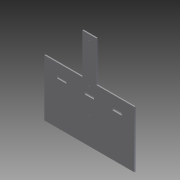
# Autodesk Inventor part: it ftront
Saved by Autodesk Inventor 2011 (Build 150239000, 239)
## iProperties
Created: 2011-08-27
Part Number: it ftront
Document SubType Name: Modeling
Designer: Matthew
Density: 1 g/cm^3
Author: Matthew
Autodesk Inventor part; units mm, degrees
(part 1 of 2)
ref_plane "YZ Plane" through (0, 0, 0) normal (1, 0, 0) x (0, 1, 0)
ref_plane "XZ Plane" through (0, 0, 0) normal (0, 1, 0) x (-1, 0, 0)
ref_plane "XY Plane" through (0, 0, 0) normal (0, 0, 1) x (1, 0, 0)
sketch "Sketch1" plane through (0, 0, 0) normal (0, 0, 1) x (1, 0, 0)
  line L0 (-143.8457, 172.4284) -> (351.4543, 172.4284)
  line L1 (351.4543, 172.4284) -> (351.4543, -716.5716)
  line L2 (351.4543, -716.5716) -> (-143.8457, -716.5716)
  line L3 (-143.8457, -716.5716) -> (-143.8457, 172.4284)
  point P0 (0, 0)
  dimension "d0" = 495.3
  dimension "d1" = 889
  constraints: 8 end point, 2 parallel, 1 horizontal, 1 perpendicular
  measures "d0" distance of L1.end L2.end
  measures "d1" distance of L0.end L1.end
extrude "Extrusion1" add sketch "Sketch1" along normal blind 6.35
sketch "Sketch2" plane through (0, 0, 6.35) normal (0, 0, 1) x (1, 0, 0)
  line L0 (-143.8457, -716.5716) -> (-105.7457, -716.5716)
  line L1 (-105.7457, -716.5716) -> (-105.7457, -640.3716)
  line L2 (-105.7457, -640.3716) -> (-143.8457, -640.3716)
  line L3 (-143.8457, -640.3716) -> (-143.8457, -716.5716)
  line L4 (-105.7457, -640.3716) -> (-124.7957, -640.3716)
  line L5 (-124.7957, -640.3716) -> (-124.7957, -659.4216)
  line L6 (-124.7957, -659.4216) -> (-105.7457, -659.4216)
  line L7 (-105.7457, -659.4216) -> (-105.7457, -640.3716)
  line L8 (351.4543, -716.5716) -> (332.4043, -716.5716)
  line L9 (332.4043, -716.5716) -> (332.4043, -659.4216)
  line L10 (332.4043, -659.4216) -> (351.4543, -659.4216)
  line L11 (351.4543, -659.4216) -> (351.4543, -716.5716)
  circle A0 centre (332.4043, -659.4216) radius 1.9812
  circle A1 centre (-124.7957, -659.4216) radius 1.9812
  point P0 (0, 0)
  dimension "d4" = 38.1
  dimension "d5" = 76.2
  dimension "d6" = 19.05
  dimension "d7" = 19.05
  dimension "d8" = 57.15
  dimension "d9" = 3.9624
  dimension "d10" = 3.9624
  constraints: 24 end point, 6 parallel, 3 horizontal, 3 perpendicular, 2 centre point, 2 coincident
  measures "d4" distance of L2.end L1.end
  measures "d5" distance of L1.end L0.end
  measures "d6" distance of L5.end L4.end
  measures "d7" distance of L9.end L10.end
  measures "d8" distance of L8.end L9.end
  measures "d9" diameter of A0
  measures "d10" diameter of A1
extrude "Extrusion2" cut sketch "Sketch2" against normal blind 6.35 contours A1 L5 L6 | L6 L5 A1 | A0 L10 L9 | L9 L10 A0
sketch "Sketch3" plane through (0, 0, 6.35) normal (0, 0, 1) x (1, 0, 0)
  line L0 (-143.8457, -716.5716) -> (-105.7457, -716.5716)
  line L1 (-105.7457, -716.5716) -> (-105.7457, -640.3716)
  line L2 (-105.7457, -640.3716) -> (-143.8457, -640.3716)
  line L3 (-143.8457, -640.3716) -> (-143.8457, -716.5716)
  line L4 (351.4543, -716.5716) -> (313.3543, -716.5716)
  line L5 (313.3543, -716.5716) -> (313.3543, -640.3716)
  line L6 (313.3543, -640.3716) -> (351.4543, -640.3716)
  line L7 (351.4543, -640.3716) -> (351.4543, -716.5716)
  line L8 (-105.7457, -716.5716) -> (313.3543, -716.5716)
  line L9 (313.3543, -716.5716) -> (313.3543, -691.1716)
  line L10 (313.3543, -691.1716) -> (-105.7457, -691.1716)
  line L11 (-105.7457, -691.1716) -> (-105.7457, -716.5716)
  line L12 (-105.7457, -691.1716) -> (313.3543, -691.1716)
  line L13 (313.3543, -691.1716) -> (313.3543, 127.9784)
  line L14 (313.3543, 127.9784) -> (-105.7457, 127.9784)
  line L15 (-105.7457, 127.9784) -> (-105.7457, -691.1716)
  point P0 (0, 0)
  dimension "d13" = 38.1
  dimension "d14" = 76.2
  dimension "d15" = 38.1
  dimension "d16" = 25.4
  dimension "d17" = 819.15
  constraints: 32 end point, 8 parallel, 4 horizontal, 4 perpendicular, 1 point on line
  measures "d13" distance of L2.end L1.end
  measures "d14" distance of L1.end L0.end
  measures "d15" distance of L5.end L6.end
  measures "d16" distance of L9.end L8.end
  measures "d17" distance of L13.end L12.end
extrude "Extrusion3" cut sketch "Sketch3" against normal blind 6.35 contours L1 L15 L14 L13 L5 L10
sketch "Sketch4" plane through (0, 0, 6.35) normal (0, 0, 1) x (1, 0, 0)
  circle A0 centre (332.4043, -659.4216) radius 1.9812 projected
  circle A1 centre (-124.7957, -659.4216) radius 1.9812 projected
  line L0 (-143.8457, -716.5716) -> (-93.0457, -716.5716)
  line L1 (-93.0457, -716.5716) -> (-93.0457, -627.6716)
  line L2 (-93.0457, -627.6716) -> (-143.8457, -627.6716)
  line L3 (-143.8457, -627.6716) -> (-143.8457, -716.5716)
  line L4 (351.4543, -716.5716) -> (300.6543, -716.5716)
  line L5 (300.6543, -716.5716) -> (300.6543, -627.6716)
  line L6 (300.6543, -627.6716) -> (351.4543, -627.6716)
  line L7 (351.4543, -627.6716) -> (351.4543, -716.5716)
  line L8 (-93.0457, -716.5716) -> (300.6543, -716.5716)
  line L9 (300.6543, -716.5716) -> (300.6543, -678.4716)
  line L10 (300.6543, -678.4716) -> (-93.0457, -678.4716)
  line L11 (-93.0457, -678.4716) -> (-93.0457, -716.5716)
  point P0 (0, 0)
  dimension "d20" = 50.8
  dimension "d21" = 88.9
  dimension "d22" = 50.8
  dimension "d23" = 88.9
  dimension "d24" = 38.1
  constraints: 24 end point, 6 parallel, 3 horizontal, 3 perpendicular, 1 point on line
  measures "d20" distance of L2.end L1.end
  measures "d21" distance of L1.end L0.end
  measures "d22" distance of L5.end L6.end
  measures "d23" distance of L4.end L5.end
  measures "d24" distance of L9.end L8.end
extrude "Extrusion4" add sketch "Sketch4" against normal blind 6.35
fillet "Fillet1" radius 6.35 8 edges at (-93.0457, -678.4716, 3.175) (-93.0457, -627.6716, 3.175) (-105.7457, -627.6716, 3.175) (300.6543, -627.6716, 3.175) (313.3543, -627.6716, 3.175) (300.6543, -678.4716, 3.175) (313.3543, 127.9784, 3.175) (-105.7457, 127.9784, 3.175)
sketch "Sketch5" plane through (0, 0, 6.35) normal (0, 0, 1) x (1, 0, 0)
  line L0 (351.4543, -716.5716) -> (-143.8457, -716.5716) projected
  line L1 (351.4543, -716.5716) -> (345.1043, -716.5716)
  line L2 (345.1043, -716.5716) -> (345.1043, -710.2216)
  line L3 (345.1043, -710.2216) -> (351.4543, -710.2216)
  line L4 (351.4543, -710.2216) -> (351.4543, -716.5716)
  line L5 (345.1043, -710.2216) -> (319.7043, -710.2216)
  line L6 (319.7043, -710.2216) -> (319.7043, -716.5716)
  line L7 (319.7043, -716.5716) -> (345.1043, -716.5716)
  line L8 (345.1043, -716.5716) -> (345.1043, -710.2216)
  line L9 (319.7043, -710.2216) -> (294.3043, -710.2216)
  line L10 (294.3043, -710.2216) -> (294.3043, -716.5716)
  line L11 (294.3043, -716.5716) -> (319.7043, -716.5716)
  line L12 (319.7043, -716.5716) -> (319.7043, -710.2216)
  line L13 (294.3043, -710.2216) -> (268.9043, -710.2216)
  line L14 (268.9043, -710.2216) -> (268.9043, -716.5716)
  line L15 (268.9043, -716.5716) -> (294.3043, -716.5716)
  line L16 (294.3043, -716.5716) -> (294.3043, -710.2216)
  line L17 (268.9043, -710.2216) -> (243.5043, -710.2216)
  line L18 (243.5043, -710.2216) -> (243.5043, -716.5716)
  line L19 (243.5043, -716.5716) -> (268.9043, -716.5716)
  line L20 (268.9043, -716.5716) -> (268.9043, -710.2216)
  line L21 (243.5043, -710.2216) -> (218.1043, -710.2216)
  line L22 (218.1043, -710.2216) -> (218.1043, -716.5716)
  line L23 (218.1043, -716.5716) -> (243.5043, -716.5716)
  line L24 (243.5043, -716.5716) -> (243.5043, -710.2216)
  line L25 (218.1043, -710.2216) -> (192.7043, -710.2216)
  line L26 (192.7043, -710.2216) -> (192.7043, -716.5716)
  line L27 (192.7043, -716.5716) -> (218.1043, -716.5716)
  line L28 (218.1043, -716.5716) -> (218.1043, -710.2216)
  line L29 (192.7043, -710.2216) -> (167.3043, -710.2216)
  line L30 (167.3043, -710.2216) -> (167.3043, -716.5716)
  line L31 (167.3043, -716.5716) -> (192.7043, -716.5716)
  line L32 (192.7043, -716.5716) -> (192.7043, -710.2216)
  line L33 (167.3043, -710.2216) -> (141.9043, -710.2216)
  line L34 (141.9043, -710.2216) -> (141.9043, -716.5716)
  line L35 (141.9043, -716.5716) -> (167.3043, -716.5716)
  line L36 (167.3043, -716.5716) -> (167.3043, -710.2216)
  line L37 (141.9043, -710.2216) -> (116.5043, -710.2216)
  line L38 (116.5043, -710.2216) -> (116.5043, -716.5716)
  line L39 (116.5043, -716.5716) -> (141.9043, -716.5716)
  line L40 (141.9043, -716.5716) -> (141.9043, -710.2216)
  line L41 (116.5043, -710.2216) -> (91.1043, -710.2216)
  line L42 (91.1043, -710.2216) -> (91.1043, -716.5716)
  line L43 (91.1043, -716.5716) -> (116.5043, -716.5716)
  line L44 (116.5043, -716.5716) -> (116.5043, -710.2216)
  line L45 (91.1043, -710.2216) -> (65.7043, -710.2216)
  line L46 (65.7043, -710.2216) -> (65.7043, -716.5716)
  line L47 (65.7043, -716.5716) -> (91.1043, -716.5716)
  line L48 (91.1043, -716.5716) -> (91.1043, -710.2216)
  line L49 (65.7043, -710.2216) -> (40.3043, -710.2216)
  line L50 (40.3043, -710.2216) -> (40.3043, -716.5716)
  line L51 (40.3043, -716.5716) -> (65.7043, -716.5716)
  line L52 (65.7043, -716.5716) -> (65.7043, -710.2216)
  line L53 (40.3043, -710.2216) -> (14.9043, -710.2216)
  line L54 (14.9043, -710.2216) -> (14.9043, -716.5716)
  line L55 (14.9043, -716.5716) -> (40.3043, -716.5716)
  line L56 (40.3043, -716.5716) -> (40.3043, -710.2216)
  line L57 (14.9043, -710.2216) -> (-10.4957, -710.2216)
  line L58 (-10.4957, -710.2216) -> (-10.4957, -716.5716)
  line L59 (-10.4957, -716.5716) -> (14.9043, -716.5716)
  line L60 (14.9043, -716.5716) -> (14.9043, -710.2216)
  line L61 (-10.4957, -710.2216) -> (-35.8957, -710.2216)
  line L62 (-35.8957, -710.2216) -> (-35.8957, -716.5716)
  line L63 (-35.8957, -716.5716) -> (-10.4957, -716.5716)
  line L64 (-10.4957, -716.5716) -> (-10.4957, -710.2216)
  line L65 (-35.8957, -710.2216) -> (-61.2957, -710.2216)
  line L66 (-61.2957, -710.2216) -> (-61.2957, -716.5716)
  line L67 (-61.2957, -716.5716) -> (-35.8957, -716.5716)
  line L68 (-35.8957, -716.5716) -> (-35.8957, -710.2216)
  line L69 (-61.2957, -710.2216) -> (-86.6957, -710.2216)
  line L70 (-86.6957, -710.2216) -> (-86.6957, -716.5716)
  line L71 (-86.6957, -716.5716) -> (-61.2957, -716.5716)
  line L72 (-61.2957, -716.5716) -> (-61.2957, -710.2216)
  line L73 (-86.6957, -710.2216) -> (-112.0957, -710.2216)
  line L74 (-112.0957, -710.2216) -> (-112.0957, -716.5716)
  line L75 (-112.0957, -716.5716) -> (-86.6957, -716.5716)
  line L76 (-86.6957, -716.5716) -> (-86.6957, -710.2216)
  line L77 (-112.0957, -710.2216) -> (-137.4957, -710.2216)
  line L78 (-137.4957, -710.2216) -> (-137.4957, -716.5716)
  line L79 (-137.4957, -716.5716) -> (-112.0957, -716.5716)
  line L80 (-112.0957, -716.5716) -> (-112.0957, -710.2216)
  point P0 (0, 0)
  dimension "d28" = 6.35
  dimension "d29" = 6.35
  dimension "d30" = 25.4
  dimension "d31" = 25.4
  dimension "d32" = 25.4
  dimension "d33" = 25.4
  dimension "d34" = 25.4
  dimension "d35" = 25.4
  dimension "d36" = 25.4
  dimension "d37" = 25.4
  dimension "d38" = 25.4
  dimension "d39" = 25.4
  dimension "d40" = 25.4
  dimension "d41" = 25.4
  dimension "d42" = 25.4
  dimension "d43" = 25.4
  dimension "d44" = 25.4
  dimension "d45" = 25.4
  dimension "d46" = 25.4
  dimension "d47" = 25.4
  dimension "d48" = 25.4
  constraints: 160 end point, 40 parallel, 20 horizontal, 20 perpendicular, 20 other
  measures "d28" distance of L2.end L3.end
  measures "d29" distance of L1.end L2.end
  measures "d30" distance of L7.end L6.end
  measures "d31" distance of L11.end L10.end
  measures "d32" distance of L15.end L14.end
  measures "d33" distance of L19.end L18.end
  measures "d34" distance of L23.end L22.end
  measures "d35" distance of L27.end L26.end
  measures "d36" distance of L31.end L30.end
  measures "d37" distance of L35.end L34.end
  measures "d38" distance of L39.end L38.end
  measures "d39" distance of L43.end L42.end
  measures "d40" distance of L47.end L46.end
  measures "d41" distance of L51.end L50.end
  measures "d42" distance of L55.end L54.end
  measures "d43" distance of L59.end L58.end
  measures "d44" distance of L63.end L62.end
  measures "d45" distance of L67.end L66.end
  measures "d46" distance of L71.end L70.end
  measures "d47" distance of L75.end L74.end
  measures "d48" distance of L79.end L78.end
extrude "Extrusion5" cut sketch "Sketch5" against normal blind 6.35 contours L0 L6 L5 L2 | L0 L14 L13 L10 | L0 L22 L21 L18 | L0 L30 L29 L26 | L0 L38 L37 L34 | L0 L46 L45 L42 | L0 L54 L53 L50 | L0 L62 L61 L58 | L0 L70 L69 L66 | L0 L78 L77 L74
sketch "Sketch6" plane through (0, 0, 6.35) normal (0, 0, 1) x (1, 0, 0)
  line L0 (-143.8457, -716.5716) -> (-143.8457, 172.4284) projected
  line L1 (-143.8457, 172.4284) -> (-137.4957, 172.4284)
  line L2 (-137.4957, 172.4284) -> (-137.4957, 121.6284)
  line L3 (-137.4957, 121.6284) -> (-143.8457, 121.6284)
  line L4 (-143.8457, 121.6284) -> (-143.8457, 172.4284)
  line L5 (-137.4957, 121.6284) -> (-143.8457, 121.6284)
  line L6 (-143.8457, 121.6284) -> (-143.8457, 70.8284)
  line L7 (-143.8457, 70.8284) -> (-137.4957, 70.8284)
  line L8 (-137.4957, 70.8284) -> (-137.4957, 121.6284)
  line L9 (-137.4957, 70.8284) -> (-143.8457, 70.8284)
  line L10 (-143.8457, 70.8284) -> (-143.8457, 20.0284)
  line L11 (-143.8457, 20.0284) -> (-137.4957, 20.0284)
  line L12 (-137.4957, 20.0284) -> (-137.4957, 70.8284)
  line L13 (-137.4957, 20.0284) -> (-143.8457, 20.0284)
  line L14 (-143.8457, 20.0284) -> (-143.8457, -30.7716)
  line L15 (-143.8457, -30.7716) -> (-137.4957, -30.7716)
  line L16 (-137.4957, -30.7716) -> (-137.4957, 20.0284)
  line L17 (-137.4957, -30.7716) -> (-143.8457, -30.7716)
  line L18 (-143.8457, -30.7716) -> (-143.8457, -81.5716)
  line L19 (-143.8457, -81.5716) -> (-137.4957, -81.5716)
  line L20 (-137.4957, -81.5716) -> (-137.4957, -30.7716)
  line L21 (-137.4957, -81.5716) -> (-143.8457, -81.5716)
  line L22 (-143.8457, -81.5716) -> (-143.8457, -132.3716)
  line L23 (-143.8457, -132.3716) -> (-137.4957, -132.3716)
  line L24 (-137.4957, -132.3716) -> (-137.4957, -81.5716)
  line L25 (-137.4957, -132.3716) -> (-143.8457, -132.3716)
  line L26 (-143.8457, -132.3716) -> (-143.8457, -183.1716)
  line L27 (-143.8457, -183.1716) -> (-137.4957, -183.1716)
  line L28 (-137.4957, -183.1716) -> (-137.4957, -132.3716)
  line L29 (-137.4957, -183.1716) -> (-143.8457, -183.1716)
  line L30 (-143.8457, -183.1716) -> (-143.8457, -233.9716)
  line L31 (-143.8457, -233.9716) -> (-137.4957, -233.9716)
  line L32 (-137.4957, -233.9716) -> (-137.4957, -183.1716)
  line L33 (-137.4957, -233.9716) -> (-143.8457, -233.9716)
  line L34 (-143.8457, -233.9716) -> (-143.8457, -284.7716)
  line L35 (-143.8457, -284.7716) -> (-137.4957, -284.7716)
  line L36 (-137.4957, -284.7716) -> (-137.4957, -233.9716)
  line L37 (-137.4957, -284.7716) -> (-143.8457, -284.7716)
  line L38 (-143.8457, -284.7716) -> (-143.8457, -335.5716)
  line L39 (-143.8457, -335.5716) -> (-137.4957, -335.5716)
  line L40 (-137.4957, -335.5716) -> (-137.4957, -284.7716)
  line L41 (-137.4957, -335.5716) -> (-143.8457, -335.5716)
  line L42 (-143.8457, -335.5716) -> (-143.8457, -386.3716)
  line L43 (-143.8457, -386.3716) -> (-137.4957, -386.3716)
  line L44 (-137.4957, -386.3716) -> (-137.4957, -335.5716)
  line L45 (-137.4957, -386.3716) -> (-143.8457, -386.3716)
  line L46 (-143.8457, -386.3716) -> (-143.8457, -437.1716)
  line L47 (-143.8457, -437.1716) -> (-137.4957, -437.1716)
  line L48 (-137.4957, -437.1716) -> (-137.4957, -386.3716)
  line L49 (-137.4957, -437.1716) -> (-143.8457, -437.1716)
  line L50 (-143.8457, -437.1716) -> (-143.8457, -487.9716)
  line L51 (-143.8457, -487.9716) -> (-137.4957, -487.9716)
  line L52 (-137.4957, -487.9716) -> (-137.4957, -437.1716)
  line L53 (-137.4957, -487.9716) -> (-143.8457, -487.9716)
  line L54 (-143.8457, -487.9716) -> (-143.8457, -538.7716)
  line L55 (-143.8457, -538.7716) -> (-137.4957, -538.7716)
  line L56 (-137.4957, -538.7716) -> (-137.4957, -487.9716)
  line L57 (-137.4957, -538.7716) -> (-143.8457, -538.7716)
  line L58 (-143.8457, -538.7716) -> (-143.8457, -589.5716)
  line L59 (-143.8457, -589.5716) -> (-137.4957, -589.5716)
  line L60 (-137.4957, -589.5716) -> (-137.4957, -538.7716)
  line L61 (-137.4957, -589.5716) -> (-143.8457, -589.5716)
  line L62 (-143.8457, -589.5716) -> (-143.8457, -640.3716)
  line L63 (-143.8457, -640.3716) -> (-137.4957, -640.3716)
  line L64 (-137.4957, -640.3716) -> (-137.4957, -589.5716)
  line L65 (-137.4957, -640.3716) -> (-143.8457, -640.3716)
  line L66 (-143.8457, -640.3716) -> (-143.8457, -691.1716)
  line L67 (-143.8457, -691.1716) -> (-137.4957, -691.1716)
  line L68 (-137.4957, -691.1716) -> (-137.4957, -640.3716)
  point P0 (0, 0)
  dimension "d51" = 50.8
  dimension "d52" = 50.8
  dimension "d53" = 50.8
  dimension "d54" = 50.8
  dimension "d55" = 50.8
  dimension "d56" = 50.8
  dimension "d57" = 50.8
  dimension "d58" = 50.8
  dimension "d59" = 50.8
  dimension "d60" = 50.8
  dimension "d61" = 50.8
  dimension "d62" = 50.8
  dimension "d63" = 50.8
  dimension "d64" = 50.8
  dimension "d65" = 50.8
  dimension "d66" = 50.8
  dimension "d67" = 50.8
  constraints: 136 end point, 34 parallel, 17 horizontal, 17 perpendicular, 17 other
  measures "d51" distance of L1.end L2.end
  measures "d52" distance of L6.end L5.end
  measures "d53" distance of L10.end L9.end
  measures "d54" distance of L14.end L13.end
  measures "d55" distance of L18.end L17.end
  measures "d56" distance of L22.end L21.end
  measures "d57" distance of L26.end L25.end
  measures "d58" distance of L30.end L29.end
  measures "d59" distance of L34.end L33.end
  measures "d60" distance of L38.end L37.end
  measures "d61" distance of L42.end L41.end
  measures "d62" distance of L46.end L45.end
  measures "d63" distance of L50.end L49.end
  measures "d64" distance of L54.end L53.end
  measures "d65" distance of L58.end L57.end
  measures "d66" distance of L62.end L61.end
  measures "d67" distance of L66.end L65.end
extrude "Extrusion6" cut sketch "Sketch6" against normal blind 6.35 contours L0 L59 L64 L63 | L0 L51 L56 L55 | L0 L43 L48 L47 | L0 L35 L40 L39 | L0 L27 L32 L31 | L0 L19 L24 L23 | L0 L11 L16 L15 | L0 L3 L8 L7
sketch "Sketch7" plane through (0, 0, 6.35) normal (0, 0, 1) x (1, 0, 0)
  line L0 (351.4543, 172.4284) -> (351.4543, -716.5716) projected
  line L1 (-137.4957, 121.6284) -> (351.4543, 121.6284)
  line L2 (-143.8457, 70.8284) -> (351.4543, 70.8284)
  line L3 (351.4543, 121.6284) -> (345.1043, 121.6284)
  line L4 (345.1043, 121.6284) -> (345.1043, 70.8284)
  line L5 (345.1043, 70.8284) -> (351.4543, 70.8284)
  line L6 (351.4543, 70.8284) -> (351.4543, 121.6284)
  line L7 (351.4543, 20.0284) -> (345.1043, 20.0284)
  line L8 (345.1043, 20.0284) -> (345.1043, -30.7716)
  line L9 (345.1043, -30.7716) -> (351.4543, -30.7716)
  line L10 (351.4543, -30.7716) -> (351.4543, 20.0284)
  line L11 (351.4543, -81.5716) -> (345.1043, -81.5716)
  line L12 (345.1043, -81.5716) -> (345.1043, -132.3716)
  line L13 (345.1043, -132.3716) -> (351.4543, -132.3716)
  line L14 (351.4543, -132.3716) -> (351.4543, -81.5716)
  line L15 (351.4543, -183.1716) -> (345.1043, -183.1716)
  line L16 (345.1043, -183.1716) -> (345.1043, -233.9716)
  line L17 (345.1043, -233.9716) -> (351.4543, -233.9716)
  line L18 (351.4543, -233.9716) -> (351.4543, -183.1716)
  line L19 (351.4543, -284.7716) -> (345.1043, -284.7716)
  line L20 (345.1043, -284.7716) -> (345.1043, -335.5716)
  line L21 (345.1043, -335.5716) -> (351.4543, -335.5716)
  line L22 (351.4543, -335.5716) -> (351.4543, -284.7716)
  line L23 (351.4543, -386.3716) -> (345.1043, -386.3716)
  line L24 (345.1043, -386.3716) -> (345.1043, -437.1716)
  line L25 (345.1043, -437.1716) -> (351.4543, -437.1716)
  line L26 (351.4543, -437.1716) -> (351.4543, -386.3716)
  line L27 (351.4543, -487.9716) -> (345.1043, -487.9716)
  line L28 (345.1043, -487.9716) -> (345.1043, -538.7716)
  line L29 (345.1043, -538.7716) -> (351.4543, -538.7716)
  line L30 (351.4543, -538.7716) -> (351.4543, -487.9716)
  line L31 (351.4543, -589.5716) -> (345.1043, -589.5716)
  line L32 (345.1043, -589.5716) -> (345.1043, -640.3716)
  line L33 (345.1043, -640.3716) -> (351.4543, -640.3716)
  line L34 (351.4543, -640.3716) -> (351.4543, -589.5716)
  point P0 (0, 0)
  constraints: 68 end point, 16 parallel, 10 horizontal, 8 perpendicular, 1 point on line, 10 other
extrude "Extrusion7" cut sketch "Sketch7" against normal blind 6.35
sketch "Sketch8" plane through (0, 0, 6.35) normal (0, 0, 1) x (1, 0, 0)
  line L0 (345.1043, -81.5716) -> (351.4543, -81.5716) projected
  line L1 (351.4543, -30.7716) -> (351.4543, -81.5716) projected
  line L2 (351.4543, -30.7716) -> (345.1043, -30.7716) projected
  line L3 (345.1043, -30.7716) -> (345.1043, 20.0284) projected
  line L4 (345.1043, 20.0284) -> (351.4543, 20.0284) projected
  line L5 (351.4543, 70.8284) -> (351.4543, 20.0284) projected
  line L6 (351.4543, 70.8284) -> (345.1043, 70.8284) projected
  line L7 (345.1043, 70.8284) -> (345.1043, 121.6284) projected
  line L8 (345.1043, 121.6284) -> (351.4543, 121.6284) projected
  line L9 (351.4543, 172.4284) -> (351.4543, 121.6284) projected
  line L10 (-143.8457, 172.4284) -> (351.4543, 172.4284) projected
  line L11 (-143.8457, 121.6284) -> (-143.8457, 172.4284) projected
  line L12 (-143.8457, 121.6284) -> (-137.4957, 121.6284) projected
  line L13 (-137.4957, 121.6284) -> (-137.4957, 70.8284) projected
  line L14 (-137.4957, 70.8284) -> (-143.8457, 70.8284) projected
  line L15 (-143.8457, 20.0284) -> (-143.8457, 70.8284) projected
  line L16 (-143.8457, 20.0284) -> (-137.4957, 20.0284) projected
  line L17 (-137.4957, 20.0284) -> (-137.4957, -30.7716) projected
  line L18 (-137.4957, -30.7716) -> (-143.8457, -30.7716) projected
  line L19 (-143.8457, -81.5716) -> (-143.8457, -30.7716) projected
  line L20 (-143.8457, -81.5716) -> (-137.4957, -81.5716) projected
  line L21 (-137.4957, -81.5716) -> (-137.4957, -132.3716) projected
  line L22 (-137.4957, -132.3716) -> (-143.8457, -132.3716) projected
  line L23 (-143.8457, -183.1716) -> (-143.8457, -132.3716) projected
  line L24 (-143.8457, -183.1716) -> (-137.4957, -183.1716) projected
  line L25 (-137.4957, -183.1716) -> (-137.4957, -233.9716) projected
  line L26 (-137.4957, -233.9716) -> (-143.8457, -233.9716) projected
  line L27 (-143.8457, -284.7716) -> (-143.8457, -233.9716) projected
  line L28 (-143.8457, -284.7716) -> (-137.4957, -284.7716) projected
  line L29 (-137.4957, -284.7716) -> (-137.4957, -335.5716) projected
  line L30 (-137.4957, -335.5716) -> (-143.8457, -335.5716) projected
  line L31 (-143.8457, -386.3716) -> (-143.8457, -335.5716) projected
  line L32 (-143.8457, -386.3716) -> (-137.4957, -386.3716) projected
  line L33 (-137.4957, -386.3716) -> (-137.4957, -437.1716) projected
  line L34 (-137.4957, -437.1716) -> (-143.8457, -437.1716) projected
  line L35 (-143.8457, -487.9716) -> (-143.8457, -437.1716) projected
  line L36 (-143.8457, -487.9716) -> (-137.4957, -487.9716) projected
  line L37 (-137.4957, -487.9716) -> (-137.4957, -538.7716) projected
  line L38 (-137.4957, -538.7716) -> (-143.8457, -538.7716) projected
  line L39 (-143.8457, -589.5716) -> (-143.8457, -538.7716) projected
  line L40 (-143.8457, -589.5716) -> (-137.4957, -589.5716) projected
  line L41 (-137.4957, -589.5716) -> (-137.4957, -640.3716) projected
  line L42 (-137.4957, -640.3716) -> (-143.8457, -640.3716) projected
  line L43 (-143.8457, -716.5716) -> (-143.8457, -640.3716) projected
  line L44 (-137.4957, -716.5716) -> (-143.8457, -716.5716) projected
  line L45 (-137.4957, -716.5716) -> (-137.4957, -710.2216) projected
  line L46 (-137.4957, -710.2216) -> (-112.0957, -710.2216) projected
  line L47 (-112.0957, -710.2216) -> (-112.0957, -716.5716) projected
  line L48 (-86.6957, -716.5716) -> (-112.0957, -716.5716) projected
  line L49 (-86.6957, -716.5716) -> (-86.6957, -710.2216) projected
  line L50 (-86.6957, -710.2216) -> (-61.2957, -710.2216) projected
  line L51 (-61.2957, -710.2216) -> (-61.2957, -716.5716) projected
  line L52 (-35.8957, -716.5716) -> (-61.2957, -716.5716) projected
  line L53 (-35.8957, -716.5716) -> (-35.8957, -710.2216) projected
  line L54 (-35.8957, -710.2216) -> (-10.4957, -710.2216) projected
  line L55 (-10.4957, -710.2216) -> (-10.4957, -716.5716) projected
  line L56 (14.9043, -716.5716) -> (-10.4957, -716.5716) projected
  line L57 (14.9043, -716.5716) -> (14.9043, -710.2216) projected
  line L58 (14.9043, -710.2216) -> (40.3043, -710.2216) projected
  line L59 (40.3043, -710.2216) -> (40.3043, -716.5716) projected
  line L60 (65.7043, -716.5716) -> (40.3043, -716.5716) projected
  line L61 (65.7043, -716.5716) -> (65.7043, -710.2216) projected
  line L62 (65.7043, -710.2216) -> (91.1043, -710.2216) projected
  line L63 (91.1043, -710.2216) -> (91.1043, -716.5716) projected
  line L64 (116.5043, -716.5716) -> (91.1043, -716.5716) projected
  line L65 (116.5043, -716.5716) -> (116.5043, -710.2216) projected
  line L66 (116.5043, -710.2216) -> (141.9043, -710.2216) projected
  line L67 (141.9043, -710.2216) -> (141.9043, -716.5716) projected
  line L68 (167.3043, -716.5716) -> (141.9043, -716.5716) projected
  line L69 (167.3043, -716.5716) -> (167.3043, -710.2216) projected
  line L70 (167.3043, -710.2216) -> (192.7043, -710.2216) projected
  line L71 (192.7043, -710.2216) -> (192.7043, -716.5716) projected
  line L72 (218.1043, -716.5716) -> (192.7043, -716.5716) projected
  line L73 (218.1043, -716.5716) -> (218.1043, -710.2216) projected
  line L74 (218.1043, -710.2216) -> (243.5043, -710.2216) projected
  line L75 (243.5043, -710.2216) -> (243.5043, -716.5716) projected
  line L76 (268.9043, -716.5716) -> (243.5043, -716.5716) projected
  line L77 (268.9043, -716.5716) -> (268.9043, -710.2216) projected
  line L78 (268.9043, -710.2216) -> (294.3043, -710.2216) projected
  line L79 (294.3043, -710.2216) -> (294.3043, -716.5716) projected
  line L80 (319.7043, -716.5716) -> (294.3043, -716.5716) projected
  line L81 (319.7043, -716.5716) -> (319.7043, -710.2216) projected
  line L82 (319.7043, -710.2216) -> (345.1043, -710.2216) projected
  line L83 (345.1043, -710.2216) -> (345.1043, -716.5716) projected
  line L84 (351.4543, -716.5716) -> (345.1043, -716.5716) projected
  line L85 (351.4543, -640.3716) -> (351.4543, -716.5716) projected
  line L86 (351.4543, -640.3716) -> (345.1043, -640.3716) projected
  line L87 (345.1043, -640.3716) -> (345.1043, -589.5716) projected
  line L88 (345.1043, -589.5716) -> (351.4543, -589.5716) projected
  line L89 (351.4543, -538.7716) -> (351.4543, -589.5716) projected
  line L90 (351.4543, -538.7716) -> (345.1043, -538.7716) projected
  line L91 (345.1043, -538.7716) -> (345.1043, -487.9716) projected
  line L92 (345.1043, -487.9716) -> (351.4543, -487.9716) projected
  line L93 (351.4543, -437.1716) -> (351.4543, -487.9716) projected
  line L94 (351.4543, -437.1716) -> (345.1043, -437.1716) projected
  line L95 (345.1043, -437.1716) -> (345.1043, -386.3716) projected
  line L96 (345.1043, -386.3716) -> (351.4543, -386.3716) projected
  line L97 (351.4543, -335.5716) -> (351.4543, -386.3716) projected
  line L98 (351.4543, -335.5716) -> (345.1043, -335.5716) projected
  line L99 (345.1043, -335.5716) -> (345.1043, -284.7716) projected
  line L100 (345.1043, -284.7716) -> (351.4543, -284.7716) projected
  line L101 (351.4543, -233.9716) -> (351.4543, -284.7716) projected
  line L102 (351.4543, -233.9716) -> (345.1043, -233.9716) projected
  line L103 (345.1043, -233.9716) -> (345.1043, -183.1716) projected
  line L104 (345.1043, -183.1716) -> (351.4543, -183.1716) projected
  line L105 (351.4543, -132.3716) -> (351.4543, -183.1716) projected
  line L106 (351.4543, -132.3716) -> (345.1043, -132.3716) projected
  line L107 (345.1043, -132.3716) -> (345.1043, -81.5716) projected
  line L108 (313.3543, 121.6284) -> (313.3543, -621.3216) projected
  line L109 (-137.4957, -716.5716) -> (345.1043, -716.5716)
  point P0 (0, 0)
  constraints: 2 end point, 1 perpendicular
extrude "Extrusion8" add sketch "Sketch8" against normal blind 6.35 contours L109 L81 L82 L83 | L109 L77 L78 L79 | L109 L73 L74 L75 | L109 L69 L70 L71 | L109 L65 L66 L67 | L109 L61 L62 L63 | L109 L57 L58 L59 | L109 L53 L54 L55 | L109 L49 L50 L51 | L109 L45 L46 L47
sketch "Sketch9" plane through (0, 0, 6.35) normal (0, 0, 1) x (1, 0, 0)
  line L0 (351.4543, -716.5716) -> (-143.8457, -716.5716) projected
  line L1 (-143.8457, -716.5716) -> (-124.7957, -716.5716)
  line L2 (-124.7957, -716.5716) -> (-124.7957, -710.2216)
  line L3 (-124.7957, -710.2216) -> (-143.8457, -710.2216)
  line L4 (-143.8457, -710.2216) -> (-143.8457, -716.5716)
  line L5 (351.4543, -716.5716) -> (332.4043, -716.5716)
  line L6 (332.4043, -716.5716) -> (332.4043, -710.2216)
  line L7 (332.4043, -710.2216) -> (351.4543, -710.2216)
  line L8 (351.4543, -710.2216) -> (351.4543, -716.5716)
  line L9 (-124.7957, -710.2216) -> (-73.9957, -710.2216)
  line L10 (-73.9957, -710.2216) -> (-73.9957, -716.5716)
  line L11 (-73.9957, -716.5716) -> (-124.7957, -716.5716)
  line L12 (-124.7957, -716.5716) -> (-124.7957, -710.2216)
  line L13 (-73.9957, -710.2216) -> (-23.1957, -710.2216)
  line L14 (-23.1957, -710.2216) -> (-23.1957, -716.5716)
  line L15 (-23.1957, -716.5716) -> (-73.9957, -716.5716)
  line L16 (-73.9957, -716.5716) -> (-73.9957, -710.2216)
  line L17 (-23.1957, -710.2216) -> (27.6043, -710.2216)
  line L18 (27.6043, -710.2216) -> (27.6043, -716.5716)
  line L19 (27.6043, -716.5716) -> (-23.1957, -716.5716)
  line L20 (-23.1957, -716.5716) -> (-23.1957, -710.2216)
  line L21 (27.6043, -710.2216) -> (78.4043, -710.2216)
  line L22 (78.4043, -710.2216) -> (78.4043, -716.5716)
  line L23 (78.4043, -716.5716) -> (27.6043, -716.5716)
  line L24 (27.6043, -716.5716) -> (27.6043, -710.2216)
  line L25 (78.4043, -716.5716) -> (129.2043, -716.5716)
  line L26 (129.2043, -716.5716) -> (129.2043, -710.2216)
  line L27 (129.2043, -710.2216) -> (78.4043, -710.2216)
  line L28 (78.4043, -710.2216) -> (78.4043, -716.5716)
  line L29 (129.2043, -710.2216) -> (180.0043, -710.2216)
  line L30 (180.0043, -710.2216) -> (180.0043, -716.5716)
  line L31 (180.0043, -716.5716) -> (129.2043, -716.5716)
  line L32 (129.2043, -716.5716) -> (129.2043, -710.2216)
  line L33 (180.0043, -716.5716) -> (230.8043, -716.5716)
  line L34 (230.8043, -716.5716) -> (230.8043, -710.2216)
  line L35 (230.8043, -710.2216) -> (180.0043, -710.2216)
  line L36 (180.0043, -710.2216) -> (180.0043, -716.5716)
  line L37 (230.8043, -710.2216) -> (281.6043, -710.2216)
  line L38 (281.6043, -710.2216) -> (281.6043, -716.5716)
  line L39 (281.6043, -716.5716) -> (230.8043, -716.5716)
  line L40 (230.8043, -716.5716) -> (230.8043, -710.2216)
  line L41 (281.6043, -710.2216) -> (332.4043, -710.2216)
  line L42 (332.4043, -710.2216) -> (332.4043, -716.5716)
  line L43 (332.4043, -716.5716) -> (281.6043, -716.5716)
  line L44 (281.6043, -716.5716) -> (281.6043, -710.2216)
  point P0 (0, 0)
  dimension "d74" = 19.05
  dimension "d75" = 6.35
  dimension "d76" = 19.05
  dimension "d77" = 6.35
  dimension "d78" = 50.8
  dimension "d79" = 50.8
  dimension "d80" = 50.8
  dimension "d81" = 50.8
  dimension "d82" = 50.8
  dimension "d83" = 50.8
  dimension "d84" = 50.8
  dimension "d85" = 50.8
  constraints: 88 end point, 22 parallel, 11 horizontal, 11 perpendicular, 6 point on line
  measures "d74" distance of L3.end L2.end
  measures "d75" distance of L2.end L1.end
  measures "d76" distance of L6.end L7.end
  measures "d77" distance of L5.end L6.end
  measures "d78" distance of L10.end L11.end
  measures "d79" distance of L14.end L15.end
  measures "d80" distance of L18.end L19.end
  measures "d81" distance of L22.end L23.end
  measures "d82" distance of L27.end L26.end
  measures "d83" distance of L30.end L31.end
  measures "d84" distance of L35.end L34.end
  measures "d85" distance of L38.end L39.end
extrude "Extrusion9" cut sketch "Sketch9" against normal blind 6.35 contours L0 L38 L41 L6 | L0 L14 L17 L18
sketch "Sketch10" plane through (0, 0, 6.35) normal (0, 0, 1) x (1, 0, 0)
  line L0 (281.6043, -716.5716) -> (27.6043, -716.5716) projected
  line L1 (-23.1957, -716.5716) -> (-143.8457, -716.5716) projected
  line L2 (-23.1957, -716.5716) -> (-73.9957, -716.5716)
  line L3 (-73.9957, -716.5716) -> (-73.9957, -710.2216)
  line L4 (-73.9957, -710.2216) -> (-23.1957, -710.2216)
  line L5 (-23.1957, -710.2216) -> (-23.1957, -716.5716)
  line L6 (-73.9957, -710.2216) -> (-124.7957, -710.2216)
  line L7 (-124.7957, -710.2216) -> (-124.7957, -716.5716)
  line L8 (-124.7957, -716.5716) -> (-73.9957, -716.5716)
  line L9 (-73.9957, -716.5716) -> (-73.9957, -710.2216)
  line L10 (27.6043, -710.2216) -> (78.4043, -710.2216)
  line L11 (78.4043, -710.2216) -> (78.4043, -716.5716)
  line L12 (78.4043, -716.5716) -> (27.6043, -716.5716)
  line L13 (27.6043, -716.5716) -> (27.6043, -710.2216)
  line L14 (78.4043, -710.2216) -> (129.2043, -710.2216)
  line L15 (129.2043, -710.2216) -> (129.2043, -716.5716)
  line L16 (129.2043, -716.5716) -> (78.4043, -716.5716)
  line L17 (78.4043, -716.5716) -> (78.4043, -710.2216)
  point P0 (0, 0)
  dimension "d88" = 50.8
  dimension "d89" = 50.8
  dimension "d90" = 50.8
  dimension "d91" = 50.8
  constraints: 32 end point, 8 parallel, 4 horizontal, 4 perpendicular, 3 point on line
  measures "d88" distance of L3.end L4.end
  measures "d89" distance of L8.end L7.end
  measures "d90" distance of L11.end L12.end
  measures "d91" distance of L15.end L16.end
extrude "Extrusion10" cut sketch "Sketch10" against normal blind 6.35 contours L0 L11 L14 L15 | L1 L7 L6 L3
sketch "Sketch11" plane through (0, 0, 6.35) normal (0, 0, 1) x (1, 0, 0)
  line L0 (281.6043, -716.5716) -> (129.2043, -716.5716) projected
  line L1 (129.2043, -710.2216) -> (180.0043, -710.2216)
  line L2 (180.0043, -710.2216) -> (180.0043, -716.5716)
  line L3 (180.0043, -716.5716) -> (129.2043, -716.5716)
  line L4 (129.2043, -716.5716) -> (129.2043, -710.2216)
  line L5 (180.0043, -710.2216) -> (230.8043, -710.2216)
  line L6 (230.8043, -710.2216) -> (230.8043, -716.5716)
  line L7 (230.8043, -716.5716) -> (180.0043, -716.5716)
  line L8 (180.0043, -716.5716) -> (180.0043, -710.2216)
  point P0 (0, 0)
  dimension "d94" = 50.8
  dimension "d95" = 50.8
  constraints: 16 end point, 4 parallel, 2 horizontal, 2 perpendicular, 2 point on line
  measures "d94" distance of L2.end L3.end
  measures "d95" distance of L6.end L7.end
extrude "Extrusion11" cut sketch "Sketch11" against normal blind 6.35 contours L0 L2 L5 L6
sketch "Sketch12" plane through (0, 0, 6.35) normal (0, 0, 1) x (1, 0, 0)
  line L0 (-143.8457, 172.4284) -> (351.4543, 172.4284) projected
  line L1 (-143.8457, 172.4284) -> (-124.7957, 172.4284)
  line L2 (-124.7957, 172.4284) -> (-124.7957, 166.0784)
  line L3 (-124.7957, 166.0784) -> (-143.8457, 166.0784)
  line L4 (-143.8457, 166.0784) -> (-143.8457, 172.4284)
  line L5 (-124.7957, 172.4284) -> (-73.9957, 172.4284)
  line L6 (-73.9957, 172.4284) -> (-73.9957, 166.0784)
  line L7 (-73.9957, 166.0784) -> (-124.7957, 166.0784)
  line L8 (-124.7957, 166.0784) -> (-124.7957, 172.4284)
  line L9 (-73.9957, 166.0784) -> (-23.1957, 166.0784)
  line L10 (-23.1957, 166.0784) -> (-23.1957, 172.4284)
  line L11 (-23.1957, 172.4284) -> (-73.9957, 172.4284)
  line L12 (-73.9957, 172.4284) -> (-73.9957, 166.0784)
  line L13 (-23.1957, 172.4284) -> (27.6043, 172.4284)
  line L14 (27.6043, 172.4284) -> (27.6043, 166.0784)
  line L15 (27.6043, 166.0784) -> (-23.1957, 166.0784)
  line L16 (-23.1957, 166.0784) -> (-23.1957, 172.4284)
  line L17 (27.6043, 166.0784) -> (78.4043, 166.0784)
  line L18 (78.4043, 166.0784) -> (78.4043, 172.4284)
  line L19 (78.4043, 172.4284) -> (27.6043, 172.4284)
  line L20 (27.6043, 172.4284) -> (27.6043, 166.0784)
  line L21 (78.4043, 172.4284) -> (129.2043, 172.4284)
  line L22 (129.2043, 172.4284) -> (129.2043, 166.0784)
  line L23 (129.2043, 166.0784) -> (78.4043, 166.0784)
  line L24 (78.4043, 166.0784) -> (78.4043, 172.4284)
  line L25 (129.2043, 166.0784) -> (180.0043, 166.0784)
  line L26 (180.0043, 166.0784) -> (180.0043, 172.4284)
  line L27 (180.0043, 172.4284) -> (129.2043, 172.4284)
  line L28 (129.2043, 172.4284) -> (129.2043, 166.0784)
  line L29 (180.0043, 172.4284) -> (230.8043, 172.4284)
  line L30 (230.8043, 172.4284) -> (230.8043, 166.0784)
  line L31 (230.8043, 166.0784) -> (180.0043, 166.0784)
  line L32 (180.0043, 166.0784) -> (180.0043, 172.4284)
  line L33 (230.8043, 166.0784) -> (281.6043, 166.0784)
  line L34 (281.6043, 166.0784) -> (281.6043, 172.4284)
  line L35 (281.6043, 172.4284) -> (230.8043, 172.4284)
  line L36 (230.8043, 172.4284) -> (230.8043, 166.0784)
  line L37 (281.6043, 172.4284) -> (332.4043, 172.4284)
  line L38 (332.4043, 172.4284) -> (332.4043, 166.0784)
  line L39 (332.4043, 166.0784) -> (281.6043, 166.0784)
  line L40 (281.6043, 166.0784) -> (281.6043, 172.4284)
  point P0 (0, 0)
  dimension "d98" = 6.35
  constraints: 80 end point, 20 parallel, 10 horizontal, 10 perpendicular, 4 point on line
  measures "d98" distance of L1.end L2.end
extrude "Extrusion12" cut sketch "Sketch12" against normal blind 6.35 contours L0 L6 L7 L2 | L0 L14 L15 L10 | L0 L22 L23 L18 | L0 L30 L31 L26 | L0 L38 L39 L34
sketch "Sketch13" plane through (0, 0, 6.35) normal (0, 0, 1) x (1, 0, 0)
  line L0 (-105.7457, -621.3216) -> (-105.7457, 121.6284) projected
  line L1 (313.3543, 121.6284) -> (313.3543, -621.3216) projected
  line L2 (-124.7957, -710.2216) -> (-73.9957, -710.2216) projected
  line L3 (-105.7457, -710.2216) -> (-105.7457, -481.6216)
  line L4 (-105.7457, -481.6216) -> (313.3543, -481.6216)
  line L5 (-105.7457, -481.6216) -> (-105.7457, -468.9216)
  line L6 (-105.7457, -468.9216) -> (313.3543, -468.9216)
  line L7 (313.3543, -468.9216) -> (313.3543, -487.9716)
  line L8 (313.3543, -487.9716) -> (-105.7457, -487.9716)
  line L9 (-105.7457, -487.9716) -> (-105.7457, -468.9216)
  point P0 (0, 0)
  dimension "d101" = 228.6
  dimension "d102" = 12.7
  dimension "d103" = 19.05
  constraints: 14 end point, 5 point on line, 2 parallel, 2 perpendicular, 1 horizontal
  measures "d101" distance of L3.start L3.end
  measures "d102" distance of L3.end L5.end
  measures "d103" distance of L6.end L7.end
extrude "Extrusion13" add sketch "Sketch13" against normal blind 25.4
sketch "Sketch14" plane through (-105.7457, -468.9216, 6.35) normal (0, 1, 0) x (1, 0, 0)
  line L0 (0, 25.4) -> (419.1, 25.4)
  line L1 (419.1, 25.4) -> (419.1, 6.35)
  line L2 (419.1, 6.35) -> (0, 6.35)
  line L3 (0, 6.35) -> (0, 25.4)
  point P0 (105.7457, 6.35)
  constraints: 8 end point, 2 parallel, 1 horizontal, 1 perpendicular
extrude "Extrusion14" cut sketch "Sketch14" against normal blind 25.4
sketch "Sketch15" plane through (0, 0, 6.35) normal (0, 0, 1) x (1, 0, 0)
  line L0 (313.3543, -468.9216) -> (-105.7457, -468.9216) projected
  line L1 (-105.7457, -468.9216) -> (129.2043, -468.9216)
  line L2 (129.2043, -468.9216) -> (129.2043, -475.2716)
  line L3 (129.2043, -475.2716) -> (78.4043, -475.2716)
  line L4 (78.4043, -475.2716) -> (78.4043, -481.6216)
  line L5 (78.4043, -481.6216) -> (129.2043, -481.6216)
  line L6 (129.2043, -481.6216) -> (129.2043, -475.2716)
  line L7 (205.4043, -481.6216) -> (230.8043, -481.6216)
  line L8 (230.8043, -481.6216) -> (230.8043, -475.2716)
  line L9 (230.8043, -475.2716) -> (205.4043, -475.2716)
  line L10 (205.4043, -475.2716) -> (205.4043, -481.6216)
  line L11 (230.8043, -475.2716) -> (281.6043, -475.2716)
  line L12 (281.6043, -475.2716) -> (281.6043, -481.6216)
  line L13 (281.6043, -481.6216) -> (230.8043, -481.6216)
  line L14 (230.8043, -481.6216) -> (230.8043, -475.2716)
  line L15 (78.4043, -475.2716) -> (-23.1957, -475.2716)
  line L16 (-23.1957, -475.2716) -> (-23.1957, -481.6216)
  line L17 (-23.1957, -481.6216) -> (78.4043, -481.6216)
  line L18 (78.4043, -481.6216) -> (78.4043, -475.2716)
  line L19 (-23.1957, -475.2716) -> (-73.9957, -475.2716)
  line L20 (-73.9957, -475.2716) -> (-73.9957, -481.6216)
  line L21 (-73.9957, -481.6216) -> (-23.1957, -481.6216)
  line L22 (-23.1957, -481.6216) -> (-23.1957, -475.2716)
  point P0 (0, 0)
  dimension "d108" = 234.95
  dimension "d109" = 6.35
  dimension "d110" = 50.8
  dimension "d111" = 6.35
  dimension "d112" = 50.8
  dimension "d113" = 101.6
  dimension "d114" = 50.8
  constraints: 44 end point, 10 parallel, 6 perpendicular, 5 horizontal, 1 point on line
  measures "d108" distance of L0.end L1.end
  measures "d109" distance of L1.end L2.end
  measures "d110" distance of L5.end L4.end
  measures "d111" distance of L4.end L3.end
  measures "d112" distance of L12.end L13.end
  measures "d113" distance of L17.end L16.end
  measures "d114" distance of L21.end L20.end
extrude "Extrusion15" cut sketch "Sketch15" against normal blind 25.4 contours L6 L5 L4 L3 | L16 L21 L20 L19 | L8 L11 L12 L13
sketch "Sketch16" plane through (0, 0, 6.35) normal (0, 0, 1) x (1, 0, 0)
  line L0 (-105.7457, -468.9216) -> (-105.7457, 121.6284) projected
  arc A0 (-99.3957, 127.9784) -> (-105.7457, 121.6284) centre (-99.3957, 121.6284) ccw projected
  line L1 (-99.3957, 127.9784) -> (307.0043, 127.9784) projected
  arc A1 (313.3543, 121.6284) -> (307.0043, 127.9784) centre (307.0043, 121.6284) ccw projected
  line L2 (313.3543, 121.6284) -> (313.3543, -468.9216) projected
  line L3 (313.3543, -468.9216) -> (-105.7457, -468.9216) projected
  line L4 (-105.7457, -487.9716) -> (313.3543, -487.9716) projected
  line L5 (313.3543, -487.9716) -> (313.3543, -621.3216) projected
  arc A2 (307.0043, -627.6716) -> (313.3543, -621.3216) centre (307.0043, -621.3216) ccw projected
  arc A3 (307.0043, -627.6716) -> (300.6543, -634.0216) centre (307.0043, -634.0216) ccw projected
  line L6 (300.6543, -634.0216) -> (300.6543, -672.1216) projected
  arc A4 (294.3043, -678.4716) -> (300.6543, -672.1216) centre (294.3043, -672.1216) ccw projected
  line L7 (294.3043, -678.4716) -> (-86.6957, -678.4716) projected
  arc A5 (-93.0457, -672.1216) -> (-86.6957, -678.4716) centre (-86.6957, -672.1216) ccw projected
  line L8 (-93.0457, -672.1216) -> (-93.0457, -634.0216) projected
  arc A6 (-93.0457, -634.0216) -> (-99.3957, -627.6716) centre (-99.3957, -634.0216) ccw projected
  arc A7 (-105.7457, -621.3216) -> (-99.3957, -627.6716) centre (-99.3957, -621.3216) ccw projected
  line L9 (-105.7457, -621.3216) -> (-105.7457, -487.9716) projected
  point P0 (0, 0)
extrude "Extrusion16" add sketch "Sketch16" against normal blind 6.35
sketch "Sketch17" plane through (0, 0, 6.35) normal (0, 0, 1) x (1, 0, 0)
  circle A0 centre (332.4043, -659.4216) radius 1.9812 projected
  circle A1 centre (-124.7957, -659.4216) radius 1.9812 projected
  point P0 (0, 0)
extrude "Extrusion17" add sketch "Sketch17" against normal blind 6.35
sketch "Sketch18" plane through (0, 0, 6.35) normal (0, 0, 1) x (1, 0, 0)
  line L0 (-143.8457, -716.5716) -> (-131.1457, -716.5716)
  line L1 (-131.1457, -716.5716) -> (-131.1457, -653.0716)
  line L2 (-131.1457, -653.0716) -> (-143.8457, -653.0716)
  line L3 (-143.8457, -653.0716) -> (-143.8457, -716.5716)
  line L4 (351.4543, -716.5716) -> (338.7543, -716.5716)
  line L5 (338.7543, -716.5716) -> (338.7543, -653.0716)
  line L6 (338.7543, -653.0716) -> (351.4543, -653.0716)
  line L7 (351.4543, -653.0716) -> (351.4543, -716.5716)
  circle A0 centre (-131.1457, -653.0716) radius 1.9812
  circle A1 centre (338.7543, -653.0716) radius 1.9812
  point P0 (0, 0)
  dimension "d121" = 12.7
  dimension "d122" = 63.5
  dimension "d123" = 12.7
  dimension "d124" = 63.5
  dimension "d125" = 3.9624
  dimension "d126" = 3.9624
  constraints: 16 end point, 4 parallel, 2 centre point, 2 coincident, 2 horizontal, 2 perpendicular
  measures "d121" distance of L2.end L1.end
  measures "d122" distance of L1.end L0.end
  measures "d123" distance of L5.end L6.end
  measures "d124" distance of L4.end L5.end
  measures "d125" diameter of A0
  measures "d126" diameter of A1
extrude "Extrusion18" cut sketch "Sketch18" against normal blind 6.35 contours A0 L2 L1 | L1 L2 A0 | A1 L6 L5 | L5 L6 A1
sketch "Sketch19" plane through (0, 0, 0) normal (0, 0, -1) x (-1, 0, 0)
  line L0 (-281.6043, -475.2716) -> (-230.8043, -475.2716)
  line L1 (-230.8043, -475.2716) -> (-230.8043, -468.9216)
  line L2 (-230.8043, -468.9216) -> (-281.6043, -468.9216)
  line L3 (-281.6043, -468.9216) -> (-281.6043, -475.2716)
  line L4 (-129.2043, -475.2716) -> (-78.4043, -475.2716)
  line L5 (-78.4043, -475.2716) -> (-78.4043, -468.9216)
  line L6 (-78.4043, -468.9216) -> (-129.2043, -468.9216)
  line L7 (-129.2043, -468.9216) -> (-129.2043, -475.2716)
  line L8 (23.1957, -475.2716) -> (73.9957, -475.2716)
  line L9 (73.9957, -475.2716) -> (73.9957, -468.9216)
  line L10 (73.9957, -468.9216) -> (23.1957, -468.9216)
  line L11 (23.1957, -468.9216) -> (23.1957, -475.2716)
  point P0 (0, 0)
  dimension "d129" = 6.35
  constraints: 24 end point, 6 parallel, 3 horizontal, 3 perpendicular
  measures "d129" distance of L1.end L0.end
extrude "Extrusion19" cut sketch "Sketch19" against normal blind 25.4
sketch "Sketch20" plane through (0, 0, 6.35) normal (0, 0, 1) x (1, 0, 0)
  line L0 (-23.1957, -468.9216) -> (-23.1957, -481.6216) projected
  line L1 (129.2043, -481.6216) -> (78.4043, -481.6216) projected
  line L2 (-23.1957, -475.2716) -> (-23.1957, -640.3716)
  line L3 (-23.1957, -640.3716) -> (-5.4157, -640.3716)
  line L4 (-5.4157, -640.3716) -> (-5.4157, -577.1256)
  line L5 (-5.4157, -640.3716) -> (-5.4157, -437.1716)
  line L6 (-5.4157, -640.3716) -> (-5.4157, -221.2716)
  circle A0 centre (-5.4157, -577.1256) radius 2.3495
  line L7 (-5.4157, -437.1716) -> (-5.4157, -439.5211)
  circle A1 centre (-5.4157, -439.5211) radius 2.3495
  circle A2 centre (-5.4157, -221.2716) radius 2.3495
  point P0 (0, 0)
  dimension "d134" = 63.246
  dimension "d135" = 203.2
  dimension "d136" = 419.1
  dimension "d137" = 4.699
  dimension "d138" = 2.3495
  constraints: 12 end point, 3 coincident, 2 centre point, 2 perpendicular, 2 point on line, 1 midpoint, 1 vertical alignment, 2 other
  measures "d134" distance of L3.end L4.end
  measures "d135" distance of L3.end L5.end
  measures "d136" distance of L3.end L6.end
  measures "d137" diameter of A0
  measures "d138" distance of L5.end L7.end
extrude "Extrusion20" cut sketch "Sketch20" against normal blind 25.4
sketch "Sketch21" plane through (0, 0, 6.35) normal (0, 0, 1) x (1, 0, 0)
  circle A0 centre (-5.4157, -577.1256) radius 2.3495 projected
  circle A1 centre (-5.4157, -221.2716) radius 2.3495 projected
  circle A2 centre (-5.4157, -439.5211) radius 2.3495 projected
  line L0 (351.4543, -538.7716) -> (351.4543, -589.5716) projected
  line L1 (351.4543, -437.1716) -> (351.4543, -487.9716) projected
  line L2 (345.1043, -233.9716) -> (345.1043, -183.1716) projected
  line L3 (230.8043, -481.6216) -> (230.8043, -468.9216) projected
  line L4 (-5.4157, -439.5211) -> (351.4543, -439.5211)
  line L5 (-5.4157, -577.1256) -> (351.4543, -577.1256)
  line L6 (-5.4157, -221.2716) -> (345.1043, -221.2716)
  line L7 (230.8043, -475.2716) -> (213.0243, -475.2716)
  line L8 (213.0243, -475.2716) -> (213.0243, -221.2716)
  line L9 (213.0243, -475.2716) -> (213.0243, -577.1256)
  circle A3 centre (213.0243, -439.5211) radius 2.3495
  circle A4 centre (213.0243, -577.1256) radius 2.3495
  circle A5 centre (213.0243, -221.2716) radius 2.3495
  point P0 (0, 0)
  dimension "d141" = 17.78
  constraints: 12 end point, 7 point on line, 5 perpendicular, 3 centre point, 2 coincident, 1 midpoint, 1 parallel
  measures "d141" distance of L7.start L7.end
extrude "Extrusion21" cut sketch "Sketch21" against normal blind 25.4 contours A3 L8 L4 | L4 L8 A3 | L8 A3 L4 | L4 A3 L8 | L9 A4 L5 | L5 A4 | L5 A4 L9 | L6 A5 | L8 A5 L6 | L6 A5 L8
sketch "Sketch22" plane through (0, 0, 6.35) normal (0, 0, 1) x (1, 0, 0)
  circle A0 centre (-5.4157, -439.5211) radius 2.3495 projected
  line L0 (129.2043, -481.6216) -> (78.4043, -481.6216) projected
  line L1 (-5.4157, -439.5211) -> (103.8043, -439.5211)
  line L2 (103.8043, -439.5211) -> (103.8043, -574.7761)
  circle A1 centre (103.8043, -439.5211) radius 2.3495
  line L3 (103.8043, -574.7761) -> (103.8043, -577.1256)
  circle A2 centre (103.8043, -577.1256) radius 2.3495
  line L4 (103.8043, -454.4264) -> (103.8043, -221.2716)
  circle A3 centre (103.8043, -221.2716) radius 2.3495
  point P0 (0, 0)
  constraints: 8 end point, 3 centre point, 3 coincident, 2 collinear, 1 parallel, 1 perpendicular, 1 point on line
extrude "Extrusion22" cut sketch "Sketch22" against normal blind 25.4 contours A1 L4 L1 | L1 L2 A1 | L4 A1 L2 | A2 | A3
sketch "Sketch23" plane through (0, 0, 6.35) normal (0, 0, 1) x (1, 0, 0)
  line L0 (195.0893, -183.1716) -> (225.3576, -183.1716)
  line L1 (225.3576, -183.1716) -> (225.3576, -596.7458)
  line L2 (225.3576, -596.7458) -> (195.0893, -596.7458)
  line L3 (195.0893, -596.7458) -> (195.0893, -183.1716)
  point P0 (0, 0)
  constraints: 8 end point, 2 parallel, 1 horizontal, 1 perpendicular
extrude "Extrusion23" add sketch "Sketch23" against normal blind 6.35
sketch "Sketch24" plane through (0, 0, 6.35) normal (0, 0, 1) x (1, 0, 0)
  circle A0 centre (-5.4157, -577.1256) radius 2.3495 projected
  circle A1 centre (-5.4157, -221.2716) radius 2.3495 projected
  circle A2 centre (-5.4157, -439.5211) radius 2.3495 projected
  circle A3 centre (-131.1457, -653.0716) radius 1.9812 projected
  circle A4 centre (338.7543, -653.0716) radius 1.9812 projected
  point P0 (0, 0)
extrude "Extrusion24" add sketch "Sketch24" against normal blind 6.35
sketch "Sketch25" plane through (0, 0, 6.35) normal (0, 0, 1) x (1, 0, 0)
  circle A0 centre (103.8043, -221.2716) radius 2.3495 projected
  circle A1 centre (103.8043, -577.1256) radius 2.3495 projected
  circle A2 centre (103.8043, -439.5211) radius 2.3495 projected
  line L0 (78.4043, -710.2216) -> (129.2043, -710.2216) projected
  line L1 (103.8043, -577.1256) -> (103.8043, -710.2216)
  line L2 (103.8043, -716.5716) -> (103.8043, -567.9054)
  circle A3 centre (103.8043, -567.9054) radius 2.3495
  line L3 (103.8043, -567.9054) -> (103.8043, -577.1256)
  line L4 (103.8043, -439.5211) -> (103.8043, -430.3009)
  line L5 (103.8043, -221.2716) -> (103.8043, -212.0514)
  circle A4 centre (103.8043, -212.0514) radius 2.3495
  circle A5 centre (103.8043, -430.3009) radius 2.3495
  point P0 (0, 0)
  dimension "d150" = 148.6662
  dimension "d151" = 9.2202
  dimension "d152" = 9.2202
  constraints: 10 end point, 3 centre point, 3 coincident, 3 collinear, 1 midpoint, 1 point on line
  measures "d150" distance of L2.start L2.end
  measures "d151" distance of L4.start L4.end
  measures "d152" distance of L5.start L5.end
extrude "Extrusion25" cut sketch "Sketch25" against normal blind 6.35 contours A3 | A4 | A5
sketch "Sketch26" plane through (0, 0, 6.35) normal (0, 0, 1) x (1, 0, 0)
  circle A0 centre (103.8043, -221.2716) radius 2.3495 projected
  circle A1 centre (103.8043, -577.1256) radius 2.3495 projected
  circle A2 centre (103.8043, -439.5211) radius 2.3495 projected
  point P0 (0, 0)
extrude "Extrusion26" add sketch "Sketch26" against normal blind 6.35